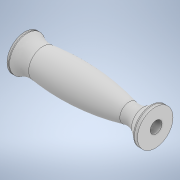
# Autodesk Inventor part: BasicHandle
Saved by Autodesk Inventor 2021 (Build 250183000, 183)
## iProperties
Created: 2021-03-22
Part Number: BasicHandle
Material: Générique
Document SubType Name: Modeling
Designer: turnb
Density: 1 g/cm^3
Appearance: Par défaut
Author: turnb
Autodesk Inventor part; units mm, degrees
ref_plane "YZ Plane" through (0, 0, 0) normal (1, 0, 0) x (0, 1, 0)
ref_plane "XZ Plane" through (0, 0, 0) normal (0, 1, 0) x (-1, 0, 0)
ref_plane "XY Plane" through (0, 0, 0) normal (0, 0, 1) x (1, 0, 0)
sketch "Esquisse1" plane through (0, 0, 0) normal (0, 0, 1) x (1, 0, 0)
  line L0 (0, 0) -> (110, 0)
  line L1 (110, 0) -> (110, 15)
  line L2 (110, 15) -> (0, 15)
  line L3 (0, 15) -> (0, 0)
  circle A0 centre (0.75, 15) radius 0.75
  circle A1 centre (108.75, 15) radius 1.25
  line L4 (108, 16) -> (100, 10)
  line L5 (1.1514, 15.6336) -> (2.1514, 15)
  arc A2 (2.1514, 15) -> (15.2922, 12.0438) centre (12.8551, 31.8947) ccw
  arc A3 (87.8865, 7.7575) -> (100, 10) centre (91.4537, 22.3272) ccw
  arc A4 (87.8865, 7.7575) -> (15.2922, 12.0438) centre (39.8874, -188.291) ccw
  point P0 (107.5, 15)
  point P1 (106.6667, 15)
  point P2 (1.5, 15)
  point P3 (0, 15)
  dimension "d2" = 1.5
  dimension "d3" = 2.5
  dimension "d0" = 110
  dimension "d1" = 15
  dimension "d4" = 10
  dimension "d5" = 8
  dimension "d6" = 1
  dimension "d7" = 20
  dimension "d8" = 15
  constraints: 12 end point, 6 point on circle, 3 centre point, 3 point on line, 3 tangent, 2 parallel, 2 vertical, 1 horizontal, 1 perpendicular, 8 other
  measures "d0" distance of L2.end L1.end
  measures "d1" distance of L0.end L1.end
  measures "d4" distance of L4.start L4.end
  measures "d5" horizontal distance of L4.start L4.end
  measures "d6" horizontal distance of L5.start L5.end
  measures "d7" radius of A2
  measures "d8" radius of A3
revolve "Révolution1" add sketch "Esquisse1" angle 360 about axis through (0, 0, 0) along (1, 0, 0) contours L3 A0 L2 A2 A4 A3 L4 A1 L1 L0
sketch "Esquisse2" plane through (0, 0, 0) normal (-1, 0, 0) x (0, 0, 1)
  point P0 (0, 0)
  point P1 (-0.7365, 0.0098)
hole "Perçage1" at (0, 0.0098, -0.7365) direction (1, 0, 0) diameter 10 end through all
move or copy body "Déplacer des corps2" bodies to move or copy 1 copy no translate (10, 0, 0)
